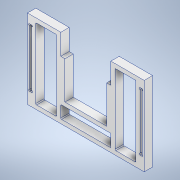
# Autodesk Inventor part: waist2
Saved by Autodesk Inventor 2022 (Build 260153000, 153)
## iProperties
Created: 2022-10-16
Part Number: waist2
Material: アルミニウム 6061
Document SubType Name: Modeling
Designer: haya
Density: 2.7 g/cm^3
Appearance: アルミニウム - フラット
Mass: 103.68 g
Surface Area: 218.198 cm^2
Volume: 38.4001 cm^3
Author: haya
Autodesk Inventor part; units mm, degrees
ref_plane "YZ Plane" through (0, 0, 0) normal (1, 0, 0) x (0, 1, 0)
ref_plane "XZ Plane" through (0, 0, 0) normal (0, 1, 0) x (-1, 0, 0)
ref_plane "XY Plane" through (0, 0, 0) normal (0, 0, 1) x (1, 0, 0)
sketch "スケッチ1" plane through (0, 0, 0) normal (0, 0, 1) x (1, 0, 0)
  line L0 (0, 0) -> (140, 0)
  line L1 (140, 0) -> (140, 95)
  line L2 (0, 95) -> (0, 0)
  line L3 (70, 94.6562) -> (70, 0) construction
  line L4 (95, 70) -> (95, 25)
  line L5 (95, 25) -> (45, 25)
  line L6 (45, 25) -> (45, 70)
  line L7 (140, 95) -> (100, 95)
  line L8 (40, 95) -> (0, 95)
  line L9 (100, 95) -> (100, 70)
  line L10 (40, 70) -> (40, 95)
  line L11 (100, 70) -> (95, 70)
  line L12 (45, 70) -> (40, 70)
  dimension "d0" = 140
  dimension "d1" = 95
  dimension "d2" = 25
  dimension "d3" = 50
  dimension "d4" = 60
  dimension "d6" = 25
  constraints: 26 end point, 6 parallel, 2 collinear, 1 horizontal, 1 midpoint, 1 perpendicular, 1 vertical, 2 other
  measures "d0" distance of L0.start L0.end
  measures "d1" distance of L2.start L0.start
  measures "d2" distance between parallel lines of L5 L0
  measures "d3" distance of L4.end L5.end
  measures "d4" distance of L9.end L10.start
  measures "d6" distance of L10.start L8.start
extrude "押し出し1" add sketch "スケッチ1" along normal blind 10
sketch "スケッチ2" plane through (0, 0, 10) normal (0, 0, 1) x (1, 0, 0)
  line L0 (0, 0) -> (140, 0) projected
  line L1 (70, 0) -> (70, 25) construction
  line L2 (95, 25) -> (45, 25) projected
  line L3 (135, 85) -> (137.5, 85)
  line L4 (137.5, 83) -> (137.5, 17)
  line L5 (137.5, 15) -> (135, 15)
  line L6 (135, 17) -> (135, 83)
  line L7 (140, 95) -> (100, 95) projected
  line L8 (140, 0) -> (140, 95) projected
  arc A0 (135, 85) -> (135, 83) centre (135, 84) ccw
  arc A1 (137.5, 83) -> (137.5, 85) centre (137.5, 84) ccw
  arc A2 (135, 17) -> (135, 15) centre (135, 16) ccw
  arc A3 (137.5, 15) -> (137.5, 17) centre (137.5, 16) ccw
  line L9 (5, 85) -> (2.5, 85)
  line L10 (2.5, 83) -> (2.5, 17)
  line L11 (2.5, 15) -> (5, 15)
  line L12 (5, 17) -> (5, 83)
  arc A4 (5, 83) -> (5, 85) centre (5, 84) ccw
  arc A5 (2.5, 85) -> (2.5, 83) centre (2.5, 84) ccw
  arc A6 (5, 15) -> (5, 17) centre (5, 16) ccw
  arc A7 (2.5, 17) -> (2.5, 15) centre (2.5, 16) ccw
  dimension "d9" = 15
  dimension "d10" = 10
  dimension "d11" = 2.5
  dimension "d12" = 2.5
  dimension "d16" = 2
  dimension "d17" = 1
  dimension "d18" = 2
  dimension "d19" = 1
  constraints: 18 end point, 16 point on circle, 12 symmetric about line, 8 centre point, 8 point on line, 2 midpoint, 2 parallel, 1 horizontal, 1 perpendicular, 1 tangent, 4 other
  measures "d9" distance between parallel lines of L5 L0
  measures "d10" distance between parallel lines of L3 L7
  measures "d11" distance between parallel lines of L8 L4
  measures "d12" distance between parallel lines of L4 L6
  measures "d16" diameter of A0
  measures "d17" radius of A1
  measures "d18" diameter of A2
  measures "d19" radius of A3
extrude "押し出し2" cut sketch "スケッチ2" against normal through all
sketch "スケッチ3" plane through (0, 0, 10) normal (0, 0, 1) x (1, 0, 0)
  line L0 (40, 20) -> (100, 20)
  line L1 (100, 20) -> (100, 5)
  line L2 (100, 5) -> (40, 5)
  line L3 (40, 5) -> (40, 20)
  arc A0 (135, 85) -> (135, 83) centre (135, 84) ccw projected
  line L4 (135, 85) -> (137.5, 85) projected
  arc A1 (137.5, 83) -> (137.5, 85) centre (137.5, 84) ccw projected
  line L5 (137.5, 83) -> (137.5, 17) projected
  arc A2 (137.5, 15) -> (137.5, 17) centre (137.5, 16) ccw projected
  line L6 (137.5, 15) -> (135, 15) projected
  arc A3 (135, 17) -> (135, 15) centre (135, 16) ccw projected
  line L7 (135, 17) -> (135, 83) projected
  arc A4 (5, 83) -> (5, 85) centre (5, 84) ccw projected
  line L8 (5, 83) -> (5, 17) projected
  arc A5 (5, 15) -> (5, 17) centre (5, 16) ccw projected
  line L9 (5, 15) -> (2.5, 15) projected
  arc A6 (2.5, 17) -> (2.5, 15) centre (2.5, 16) ccw projected
  line L10 (2.5, 17) -> (2.5, 83) projected
  arc A7 (2.5, 85) -> (2.5, 83) centre (2.5, 84) ccw projected
  line L11 (2.5, 85) -> (5, 85) projected
  line L12 (140, 0) -> (140, 95) projected
  line L13 (140, 95) -> (100, 95) projected
  line L14 (100, 95) -> (100, 70) projected
  line L15 (100, 70) -> (95, 70) projected
  line L16 (95, 70) -> (95, 25) projected
  line L17 (95, 25) -> (45, 25) projected
  line L18 (45, 25) -> (45, 70) projected
  line L19 (45, 70) -> (40, 70) projected
  line L20 (40, 70) -> (40, 95) projected
  line L21 (40, 95) -> (0, 95) projected
  line L22 (0, 95) -> (0, 0) projected
  line L23 (0, 0) -> (140, 0) projected
  line L24 (45, 25) -> (45, 70) projected
  line L25 (95, 70) -> (95, 25) projected
  line L26 (105, 90) -> (130, 90)
  line L27 (130, 90) -> (130, 5)
  line L28 (130, 5) -> (105, 5)
  line L29 (105, 5) -> (105, 90)
  line L30 (95, 25) -> (45, 25) projected
  line L31 (70, 25) -> (70, 0) construction
  line L32 (35, 90) -> (10, 90)
  line L33 (10, 90) -> (10, 5)
  line L34 (10, 5) -> (35, 5)
  line L35 (35, 5) -> (35, 90)
  dimension "d20" = 5
  dimension "d21" = 5
  dimension "d22" = 5
  dimension "d23" = 5
  dimension "d24" = 10
  dimension "d25" = 5
  dimension "d26" = 5
  constraints: 26 end point, 4 symmetric about line, 3 parallel, 2 horizontal, 2 midpoint, 1 perpendicular, 1 other
  measures "d20" distance between parallel lines of L0 L17
  measures "d21" distance between parallel lines of L23 L2
  measures "d22" distance between parallel lines of L29 L14
  measures "d23" distance between parallel lines of L26 L13
  measures "d24" distance between parallel lines of L12 L27
  measures "d25" distance between parallel lines of L28 L23
  measures "d26" distance between parallel lines of L1 L29
extrude "押し出し3" cut sketch "スケッチ3" against normal through all contours L0 L1 L2 L3 | L26 L27 L28 L29 | L35 L34 L33 L32
fillet "フィレット1" radius 1 12 edges at (35, 90, 5) (10, 90, 5) (10, 5, 5) (35, 5, 5) (40, 5, 5) (40, 20, 5) (100, 5, 5) (100, 20, 5) (130, 90, 5) (105, 90, 5) (105, 5, 5) (130, 5, 5)
